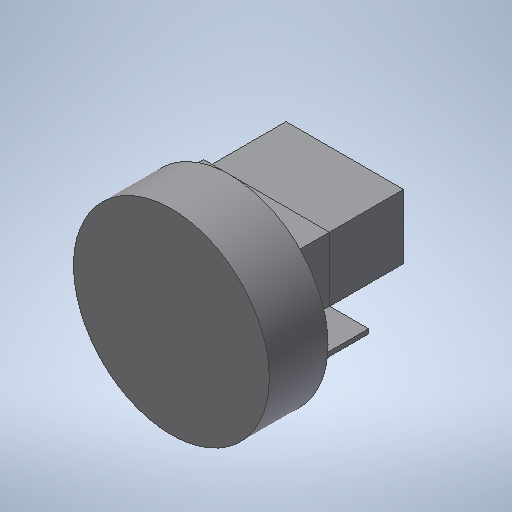
# Autodesk Inventor part: Rueda Izquierda
Saved by Autodesk Inventor 2025 (Build 290162000, 162)
## iProperties
Created: 2024-10-07
Part Number: Rueda Izquierda
Material: Generic
Document SubType Name: Modeling
Designer: feder
Density: 1 g/cm^3
Appearance: Default
Author: feder
Autodesk Inventor part; units mm, degrees
ref_plane "YZ Plane" through (0, 0, 0) normal (1, 0, 0) x (0, 1, 0)
ref_plane "XZ Plane" through (0, 0, 0) normal (0, 1, 0) x (-1, 0, 0)
ref_plane "XY Plane" through (0, 0, 0) normal (0, 0, 1) x (1, 0, 0)
sketch "Sketch1" plane through (0, 0, 0) normal (0, 0, 1) x (1, 0, 0)
  circle A0 centre (0, 0) radius 35
  dimension "d0" = 70
  constraints: 1 centre point, 1 coincident
  measures "d0" diameter of A0
extrude "Extrusion1" add sketch "Sketch1" along normal blind 21
sketch "Sketch2" plane through (0, 0, 0) normal (0, 0, -1) x (-1, 0, 0)
  circle A0 centre (0, 0) radius 7
  dimension "d3" = 14
  constraints: 1 centre point, 1 coincident
  measures "d3" diameter of A0
extrude "Extrusion2" add sketch "Sketch2" along normal blind 5
sketch "Sketch3" plane through (0, 0, -5) normal (0, 0, -1) x (-1, 0, 0)
  line L0 (-12, 11.5) -> (30, 11.5)
  line L1 (30, 11.5) -> (30, -11.5)
  line L2 (30, -11.5) -> (-12, -11.5)
  line L3 (-12, -11.5) -> (-12, 11.5)
  point P0 (0, 0)
  point P1 (30, 0)
  point P2 (-12, 0)
  dimension "d6" = 23
  dimension "d7" = 42
  dimension "d8" = 12
  constraints: 8 end point, 2 midpoint, 2 parallel, 1 horizontal, 1 horizontal alignment, 1 perpendicular
  measures "d6" distance of L0.end L1.end
  measures "d7" distance of L0.start L0.end
  measures "d8" distance of point (0, 0) point (-12, 0)
extrude "Extrusion3" add sketch "Sketch3" along normal blind 45
sketch "Sketch4" plane through (-30, 11.5, -5) normal (0, 1, 0) x (1, 0, 0)
  line L0 (42, 0) -> (0, 0) projected
  line L1 (0, 0) -> (42, 0)
  line L2 (42, 0) -> (42, 17)
  line L3 (42, 17) -> (0, 17)
  line L4 (0, 17) -> (0, 0)
  point P0 (30, -5)
  dimension "d11" = 17
  dimension "d12" = 42
  constraints: 8 end point, 2 parallel, 1 horizontal, 1 perpendicular
  measures "d11" distance of L1.end L2.end
  measures "d12" distance of L2.end L3.end
extrude "Extrusion4" add sketch "Sketch4" along normal blind 1.5
sketch "Sketch5" plane through (12, -11.5, -50) normal (1, 0, 0) x (0, 0, -1)
  line L0 (-28, 24.5) -> (-45, 24.5) projected
  line L1 (-28, 24.5) -> (-45, 24.5)
  line L2 (-45, 24.5) -> (-45, 0)
  line L3 (-45, 0) -> (-28, 0)
  line L4 (-28, 0) -> (-28, 24.5)
  point P0 (-50, 11.5)
  constraints: 8 end point, 2 parallel, 1 horizontal, 1 perpendicular
extrude "Extrusion5" add sketch "Sketch5" along normal blind 1.5
sketch "Sketch6" plane through (-30, -11.5, -50) normal (-1, 0, 0) x (0, 0, 1)
  point P0 (50, 11.5)
sketch "Sketch7" plane through (-30, -11.5, -50) normal (-1, 0, 0) x (0, 0, 1)
  line L0 (28, 23) -> (28, 24.5) projected
  line L1 (45, 0) -> (45, 24.5) projected
  line L2 (28, 24.5) -> (45, 24.5)
  line L3 (45, 24.5) -> (45, 0)
  line L4 (45, 0) -> (28, 0)
  line L5 (28, 0) -> (28, 24.5)
  point P0 (50, 11.5)
  constraints: 8 end point, 2 parallel, 1 horizontal, 1 perpendicular
extrude "Extrusion6" add sketch "Sketch7" along normal blind 1.5
sketch "Sketch8" plane through (-31.5, -11.5, -50) normal (-1, 0, 0) x (0, 0, 1)
  line L0 (45, 24.5) -> (45, 0) projected
  line L1 (28, 23) -> (28, 0) projected
  line L2 (45, 0) -> (28, 0)
  line L3 (28, 0) -> (28, 1.6)
  line L4 (28, 1.6) -> (45, 1.6)
  line L5 (45, 1.6) -> (45, 0)
  point P0 (50, 11.5)
  dimension "d19" = 1.6
  constraints: 8 end point, 2 parallel, 1 horizontal, 1 perpendicular, 1 point on line
  measures "d19" distance between parallel lines of L2 L4
extrude "Extrusion7" add sketch "Sketch8" along normal blind 14
sketch "Sketch9" plane through (13.5, -11.5, -50) normal (1, 0, 0) x (0, 0, -1)
  line L0 (-45, 0) -> (-28, 0) projected
  line L1 (-28, 23) -> (-28, 0) projected
  line L2 (-45, 0) -> (-28, 0)
  line L3 (-28, 0) -> (-28, 1.6)
  line L4 (-28, 1.6) -> (-45, 1.6)
  line L5 (-45, 1.6) -> (-45, 0)
  point P0 (-50, 11.5)
  dimension "d22" = 1.6
  constraints: 8 end point, 2 parallel, 1 horizontal, 1 perpendicular, 1 point on line
  measures "d22" distance of L4.end L0.start
extrude "Extrusion8" add sketch "Sketch9" along normal blind 14
body "Solid1"
